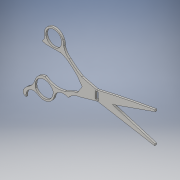
# Autodesk Inventor part: RTS Scissors
Saved by Autodesk Inventor 2016 (Build 200138000, 138)
## iProperties
Created: 2017-12-19
Part Number: RTS Scissors
Material: Generic
Document SubType Name: Modeling
Designer: student
Density: 1 g/cm^3
Appearance: Default
Author: student
Autodesk Inventor part; units mm, degrees
ref_plane "YZ Plane" through (0, 0, 0) normal (1, 0, 0) x (0, 1, 0)
ref_plane "XZ Plane" through (0, 0, 0) normal (0, 1, 0) x (-1, 0, 0)
ref_plane "XY Plane" through (0, 0, 0) normal (0, 0, 1) x (1, 0, 0)
sketch "Sketch1" plane through (0, 0, 0) normal (0, 0, 1) x (1, 0, 0)
  line L0 (-121.92, 53.34) -> (121.92, 53.34)
  line L1 (121.92, 53.34) -> (121.92, -53.34)
  line L2 (121.92, -53.34) -> (-121.92, -53.34)
  line L3 (-121.92, -53.34) -> (-121.92, 53.34)
  line L4 (-121.92, 53.34) -> (121.92, -53.34) construction
  line L5 (121.92, 53.34) -> (-121.92, -53.34) construction
  line L6 (99.0307, 67.3864) -> (98.1801, -71.8373) construction
  line L7 (98.1801, -71.8373) -> (-108.1272, -70.5768) construction
  line L8 (-108.1272, -70.5768) -> (-107.2765, 68.6469) construction
  line L9 (-107.2765, 68.6469) -> (99.0307, 67.3864) construction
  arc A0 (-78.8873, -40.6173) -> (-95.4767, -51.4852) centre (-84.9112, -49.5176) ccw
  arc A1 (-78.8873, -40.6173) -> (-56.3395, -33.0982) centre (-70.4947, -28.2175) ccw
  arc A2 (-36.1227, -22.9374) -> (-56.3395, -33.0982) centre (-42.6558, -35.1316) ccw
  arc A3 (-19.5186, -13.8085) -> (-36.1227, -22.9374) centre (-17.295, -37.5173) ccw
  arc A4 (-68.7224, -13.6289) -> (-40.5344, -17.4333) centre (-51.1537, 10.214) ccw
  arc A5 (-68.7224, -13.6289) -> (-83.4187, -26.4721) centre (-67.6747, -29.6577) ccw
  arc A6 (-92.1839, -37.2444) -> (-83.4187, -26.4721) centre (-103.1345, -19.3818) ccw
  arc A7 (-92.1839, -37.2444) -> (-99.3105, -45.0028) centre (-83.147, -52.6977) ccw
  arc A8 (-99.3105, -45.0028) -> (-95.4767, -51.4852) centre (-95.2121, -46.9539) ccw
  arc A9 (-82.2314, -34.4993) -> (-57.5296, -25.5657) centre (-70.7814, -27.5415) ccw
  arc A10 (-57.5296, -25.5657) -> (-82.2314, -34.4993) centre (-69.6152, -30.7661) ccw
  line L10 (5.4328, -6.7323) -> (-19.5186, -13.8085)
  line L11 (5.4328, -6.7323) -> (85.4483, -20.8459)
  line L12 (85.4483, -20.8459) -> (85.8807, -18.3941)
  line L13 (85.8807, -18.3941) -> (26.167, -0.0762)
  line L14 (26.167, -0.0762) -> (86.2931, 21.1025)
  line L15 (86.2931, 21.1025) -> (85.711, 23.1551)
  arc A11 (85.711, 23.1551) -> (3.7291, 6.4763) centre (298.902, -1234.5808) ccw
  line L16 (-54.4933, 26.4309) -> (-67.6017, 26.4309)
  line L17 (-67.6017, 26.4309) -> (-72.6264, 27.9793)
  line L18 (-72.6264, 27.9793) -> (-69.6152, 32.3411)
  line L19 (-69.6152, 32.3411) -> (-69.6152, 41.676)
  arc A12 (-43.7838, 43.5271) -> (-69.6152, 41.676) centre (-56.4305, 38.848) ccw
  arc A13 (-47.6138, 46.2719) -> (-67.6017, 37.0085) centre (-56.174, 38.5465) ccw
  arc A14 (-67.6017, 37.0085) -> (-47.6138, 46.2719) centre (-56.6407, 39.5536) ccw
  arc A15 (-42.5631, 37.0085) -> (-43.7838, 43.5271) centre (-53.7825, 38.2811) ccw
  arc A16 (-42.5631, 37.0085) -> (-34.9749, 24.888) centre (-24.5395, 39.8568) ccw
  line L20 (-54.4933, 26.4309) -> (-47.0393, 26.4309)
  arc A17 (-36.0743, 21.1026) -> (-47.0393, 26.4309) centre (-51.4449, 3.4184) ccw
  arc A18 (-22.5276, 8.9937) -> (-36.0743, 21.1026) centre (-88.9207, -51.6509) ccw
  arc A19 (-34.9749, 24.888) -> (-17.1938, 11.6747) centre (31.7815, 96.1512) ccw
  line L21 (-22.5276, 8.9937) -> (-16.445, 0)
  line L22 (-16.445, 0) -> (-22.747, -9.6513)
  line L23 (-22.747, -9.6513) -> (-40.5344, -17.4333)
  line L24 (-17.1938, 11.6747) -> (3.7291, 6.4763)
  line L25 (-16.445, 0) -> (3.7291, 6.4763)
  line L26 (5.4328, -6.7323) -> (26.167, -0.0762)
  line L27 (2.2389, 4.8137) -> (6.6839, 4.8137)
  line L28 (6.6839, 4.8137) -> (6.6839, -5.3463)
  line L29 (6.6839, -5.3463) -> (2.2389, -5.3463)
  line L30 (2.2389, -5.3463) -> (2.2389, 4.8137)
  line L31 (2.2389, 4.8137) -> (6.6839, -5.3463) construction
  line L32 (6.6839, 4.8137) -> (2.2389, -5.3463) construction
  point P0 (0, 0)
  point P1 (4.4614, -0.2663)
  dimension "d0" = 243.84
  dimension "d1" = 106.68
  dimension "d23" = 4.445
  dimension "d24" = 10.16
  constraints: 58 end point, 40 point on circle, 20 centre point, 6 parallel, 5 perpendicular, 4 horizontal, 4 midpoint, 2 tangent, 2 other
  measures "d0" distance of L1.end L2.end
  measures "d1" distance of L0.end L1.end
  measures "d23" distance of L28.end L29.end
  measures "d24" distance of L27.end L28.end
extrude "Extrusion2" add sketch "Sketch1" along normal blind 2.54 contours A0 A8 A7 A6 A5 A4 L23 L22 L25 A11 L15 L14 L26 L10 A3 A2 A1 | L26 L13 L12 L11 | L21 A18 A17 L20 L16 L17 L18 L19 A12 A15 A16 A19 L24 L25
body "Solid2"
